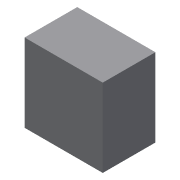
# Autodesk Inventor part: PegHead
Saved by Autodesk Inventor 2015 (Build 190159000, 159)
## iProperties
Created: 2015-03-07
Part Number: PegHead
Material: Iron, Malleable
Document SubType Name: Modeling
Designer: Jaden
Density: 7.15 g/cm^3
Appearance: Semi-Polished
Author: Jaden
Autodesk Inventor part; units mm, degrees
ref_plane "YZ Plane" through (0, 0, 0) normal (1, 0, 0) x (0, 1, 0)
ref_plane "XZ Plane" through (0, 0, 0) normal (0, 1, 0) x (-1, 0, 0)
ref_plane "XY Plane" through (0, 0, 0) normal (0, 0, 1) x (1, 0, 0)
sketch "Sketch1" plane through (0, 0, 0) normal (0, 0, 1) x (1, 0, 0)
  line L0 (0, 0) -> (3.7707, 0)
  line L1 (3.7707, 0) -> (3.7707, 3.7707)
  line L2 (3.7707, 3.7707) -> (0, 3.7707)
  line L3 (0, 3.7707) -> (0, 0)
  dimension "d2" = 3.7707
  dimension "d3" = 3.7707
  constraints: 8 end point, 2 parallel, 1 horizontal, 1 perpendicular
  measures "d2" distance of L2.end L1.end
  measures "d3" distance of L1.end L0.end
extrude "Extrusion1" add sketch "Sketch1" along normal blind 2.54
body "Solid1"
